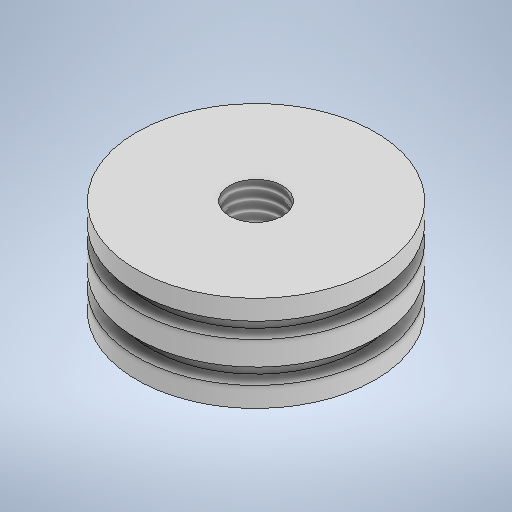
# Autodesk Inventor part: 2021
Saved by Autodesk Inventor 2025 (Build 290162010, 162A)
## iProperties
Created: 2024-05-30
Part Number: 2021
Material: Generic
Document SubType Name: Modeling
Designer: Fabri
Density: 1 g/cm^3
Appearance: Default
Author: Fabri
Autodesk Inventor part; units mm, degrees
ref_plane "YZ Plane" through (0, 0, 0) normal (1, 0, 0) x (0, 1, 0)
ref_plane "XZ Plane" through (0, 0, 0) normal (0, 1, 0) x (-1, 0, 0)
ref_plane "XY Plane" through (0, 0, 0) normal (0, 0, 1) x (1, 0, 0)
sketch "Sketch1" plane through (0, 0, 0) normal (0, 1, 0) x (-1, 0, 0)
  line L0 (0, 0) -> (15, 0)
  line L1 (15, 0) -> (15, -2.5)
  line L2 (15, -2.5) -> (13.25, -2.5)
  line L3 (13.25, -2.5) -> (13.25, -4.5)
  line L4 (13.25, -4.5) -> (15, -4.5)
  line L5 (15, -4.5) -> (15, -7.5)
  line L6 (15, -7.5) -> (13.25, -7.5)
  line L7 (13.25, -7.5) -> (13.25, -9.5)
  line L8 (13.25, -9.5) -> (15, -9.5)
  line L9 (15, -9.5) -> (15, -12)
  line L10 (15, -12) -> (0, -12)
  line L11 (0, -12) -> (0, 0)
  dimension "d0" = 2.5
  dimension "d2" = 2.5
  dimension "d3" = 2
  dimension "d4" = 2
  dimension "d7" = 12
  dimension "d8" = 26.5
  dimension "d9" = 30
  constraints: 24 end point, 8 perpendicular, 6 point on line, 1 horizontal
  measures "d0" distance between parallel lines of L10 L8
  measures "d2" distance between parallel lines of L2 L0
  measures "d3" distance of L2.end L3.end
  measures "d4" distance of L6.end L7.end
  measures "d7" distance between parallel lines of L10 L0
  measures "d8" diameter of L7 L11
  measures "d9" diameter of L9 L11
revolve "Revolution1" add sketch "Sketch1" angle 360 about axis through (0, 0, -12) along (0, 0, 1)
sketch "Sketch2" plane through (0, 0, -12) normal (0, 0, -1) x (-1, 0, 0)
  circle A0 centre (0, 0) radius 15 projected
  point P0 (0, 0)
  constraints: 1 coincident
hole "Hole1" at (0, 0, -12) direction (0, 0, 1) diameter 6.647 end through all counterbore diameter 9 counterbore depth 5 thread size "M8x1.25" class "6H" standard "ISO Metric profile"
body "Solid1"
